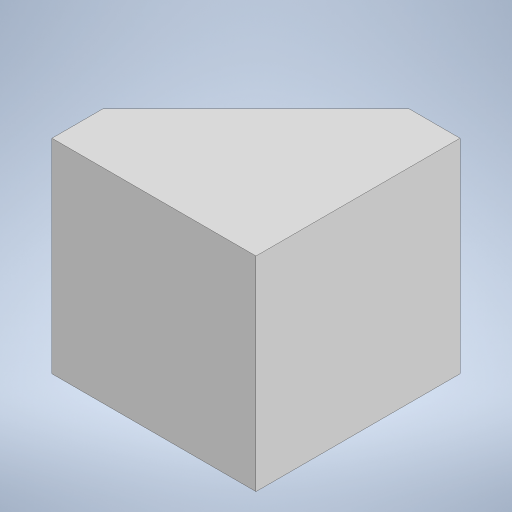
# Autodesk Inventor part: tunnel corner bracket
Saved by Autodesk Inventor 2023 (Build 270158000, 158)
## iProperties
Created: 2021-04-13
Part Number: tunnel corner bracket
Material: Generic
Document SubType Name: Modeling
Designer: KAMPFF-LAB-BEHAVIOR
Density: 1 g/cm^3
Appearance: Default
Author: KAMPFF-LAB-BEHAVIOR
Autodesk Inventor part; units mm, degrees
ref_plane "YZ Plane" through (0, 0, 0) normal (1, 0, 0) x (0, 1, 0)
ref_plane "XZ Plane" through (0, 0, 0) normal (0, 1, 0) x (-1, 0, 0)
ref_plane "XY Plane" through (0, 0, 0) normal (0, 0, 1) x (1, 0, 0)
sketch "Sketch30" plane through (0, 0, 0) normal (0, 0, 1) x (1, 0, 0)
  line L0 (0, 0) -> (-20, 0)
  line L1 (-20, 0) -> (-20, 20)
  line L2 (-20, 20) -> (0, 20)
  line L3 (0, 20) -> (0, 0)
  dimension "d101" = 20
  dimension "d102" = 20
  constraints: 8 end point, 2 parallel, 1 horizontal, 1 perpendicular
  measures "d101" distance of L1.end L2.end
  measures "d102" distance of L0.end L1.end
extrude "Extrusion22" add sketch "Sketch30" against normal blind 5
sketch "Sketch31" plane through (0, 0, 0) normal (1, 0, 0) x (0, 0, -1)
  line L0 (0, 0) -> (0, 20) projected
  line L1 (0, 0) -> (20, 0)
  line L2 (20, 0) -> (20, 20)
  line L3 (20, 20) -> (0, 20)
  line L4 (0, 20) -> (0, 0)
  dimension "d105" = 20
  constraints: 8 end point, 2 parallel, 1 horizontal, 1 perpendicular
  measures "d105" distance of L3.end L2.end
extrude "Extrusion23" add sketch "Sketch31" against normal blind 5
sketch "Sketch32" plane through (-20, 20, 0) normal (0, 1, 0) x (1, 0, 0)
  line L0 (0, 5) -> (15, 5) projected
  line L1 (15, 20) -> (15, 5) projected
  line L2 (15, 5) -> (15, 20)
  line L3 (15, 20) -> (0, 5)
  line L4 (0, 5) -> (15, 5)
  point P0 (20, 0)
  constraints: 6 end point, 1 perpendicular, 1 vertical
extrude "Extrusion24" add sketch "Sketch32" against normal blind 5
sketch "Sketch33" plane through (-20, 0, 0) normal (0, -1, 0) x (1, 0, 0)
  line L0 (0, 0) -> (0, -5) projected
  line L1 (15, -20) -> (15, -5) projected
  line L2 (0, -5) -> (15, -5)
  line L3 (15, -5) -> (15, -20)
  line L4 (0, -5) -> (15, -20) projected
  line L5 (15, -20) -> (0, -5)
  point P0 (20, 0)
  constraints: 6 end point, 2 collinear, 1 horizontal
extrude "Extrusion25" add sketch "Sketch33" against normal blind 5
body "Solid6"
